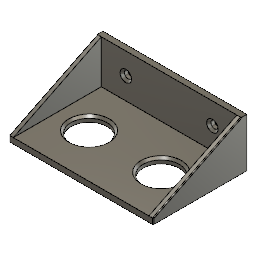
Porta_condimentos v2 (Autodesk Fusion 360 design; units mm, degrees)
Autodesk Fusion 360 part; units mm, degrees
sketch "Sketch1" plane through (0, 0, 0) normal (0, 1, 0) x (1, 0, 0)
  line L0 (0, 0) -> (0, -65)
  line L1 (0, -65) -> (100, -65)
  line L2 (100, -65) -> (100, 0)
  line L3 (100, 0) -> (0, 0)
  dimension "d1" = 65
  measures "d1" distance of L0.start
extrude "Extrude1" add sketch "Sketch1" along normal blind 4 makes body 1
sketch "Sketch2" plane through (0, 4, 0) normal (0, 1, 0) x (-1, 0, 0)
  line L0 (-100, 0) -> (0, 0)
  line L1 (0, 0) -> (0, 65)
  line L2 (0, 65) -> (-100, 65)
  line L3 (-100, 65) -> (-100, 0)
  line L4 (0, 0) -> (-100, 0)
  line L5 (-100, 0) -> (-100, 4)
  line L6 (0, 0) -> (0, 4)
  line L7 (0, 4) -> (-100, 4)
  dimension "d4" = 4
  dimension "d5" = 4
  measures "d4" distance of L0.end
  measures "d5" distance of L0.end
extrude "Extrude2" add sketch "Sketch2" along normal blind 30 contours L0 L1 L3 L4 L5 L6 L7 bodies 1
sketch "Sketch4" plane through (0, 4, 0) normal (0, 1, 0) x (-1, 0, 0)
  line L0 (-100, 4) -> (0, 4)
  line L1 (0, 4) -> (0, 65)
  line L2 (0, 65) -> (-100, 65)
  line L3 (-100, 65) -> (-100, 4)
  line L4 (-50, 4) -> (-50, 65) construction
  line L5 (-50, 34.5) -> (-25, 34.5) construction
  circle A0 centre (-25, 34.5) radius 12.5
  circle A1 centre (-75, 34.5) radius 12.5
  dimension "d8" = 25
  dimension "d9" = 25
  measures "d9" diameter of A0
sketch "Sketch6" plane through (0, 0, 0) normal (-1, 0, 0) x (0, 0, 1)
  line L0 (0, 0) -> (65, 0)
  line L1 (65, 0) -> (65, 4)
  line L2 (65, 4) -> (4, 4)
  line L3 (4, 4) -> (4, 34)
  line L4 (4, 34) -> (0, 34)
  line L5 (0, 34) -> (0, 0)
  line L6 (4, 34) -> (4, 4)
  line L7 (65, 4) -> (4, 34)
extrude "Extrude3" add sketch "Sketch6" against normal blind 3 separate body contours L2 L3 L6 L7 makes body 2
ref_plane "WorkPlane1" through (50, 19, 34.5) normal (-1, 0, 0) x (0, 0, 1)
mirror "Mirror1" about plane through (50, 19, 34.5) normal (-1, 0, 0) of bodies 2 makes body 3
extrude "Extrude4" cut sketch "Sketch4" against normal blind 30 contours A0 | A1 bodies 1
chamfer "Chamfer1" distance 1.5 angle 45 2 edges at (86.6541, 4, 39.0202) (36.6541, 4, 39.0202) on bodies 1
sketch "Sketch7" plane through (0, 0, 4) normal (0, 0, 1) x (1, 0, 0)
  line L0 (0, 4) -> (100, 4)
  line L1 (100, 4) -> (100, 34)
  line L2 (100, 34) -> (0, 34)
  line L3 (0, 34) -> (0, 4)
  line L4 (50, 34) -> (50, 19) construction
  line L5 (50, 19) -> (20, 19)
  circle A0 centre (20, 19) radius 2.5
  circle A1 centre (80, 19) radius 2.5
  dimension "d17" = 15
  dimension "d18" = 30
  dimension "d19" = 5
  measures "d17" distance of origin
  measures "d19" diameter of A0
extrude "Extrude5" cut sketch "Sketch7" against normal blind 29 contours A0 | A1 bodies 1
chamfer "Chamfer2" distance 1.5 angle 45 2 edges at (77.6692, 19.904, 4) (17.6692, 19.904, 4) on bodies 1
fillet "Fillet4" radius 0.5 4 edges at (0, 2, 65) (100, 2, 65) (0, 19, 34.5) (100, 19, 34.5) on bodies 1 2 3
combine "Combine1" operation add target body 1 tool bodies 2 3
